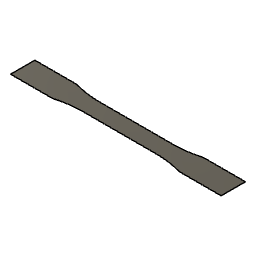
specimen_plastic_tensile_testing v3 (Autodesk Fusion 360 design; units mm, degrees)
Autodesk Fusion 360 part; units mm, degrees
sketch "Esquisse1" plane through (0, 0, 0) normal (0, 0, 1) x (1, 0, 0)
  line L0 (-28.5, 6.5) -> (0, 6.5)
  line L1 (0, 6.5) -> (0, 0) construction
  line L2 (0, 0) -> (-35.4205, 0) construction
  line L3 (-82.5, 9.5) -> (-49.6424, 9.5)
  line L4 (-35.4205, 0) -> (-82.5, 0) construction
  line L5 (-82.5, 0) -> (-82.5, 9.5)
  arc A0 (-49.6424, 9.5) -> (-28.5, 6.5) centre (-28.5, 82.5) ccw
  line L6 (-28.5, -6.5) -> (0, -6.5)
  arc A1 (-28.5, -6.5) -> (-49.6424, -9.5) centre (-28.5, -82.5) ccw
  line L7 (-82.5, -9.5) -> (-49.6424, -9.5)
  line L8 (-82.5, 0) -> (-82.5, -9.5)
  arc A2 (49.6424, -9.5) -> (28.5, -6.5) centre (28.5, -82.5) ccw
  line L9 (28.5, -6.5) -> (0, -6.5)
  line L10 (82.5, -9.5) -> (49.6424, -9.5)
  line L11 (82.5, 0) -> (82.5, -9.5)
  line L12 (82.5, 0) -> (82.5, 9.5)
  line L13 (82.5, 9.5) -> (49.6424, 9.5)
  arc A3 (28.5, 6.5) -> (49.6424, 9.5) centre (28.5, 82.5) ccw
  line L14 (28.5, 6.5) -> (0, 6.5)
  dimension "d1" = 28.5
  dimension "d9" = 6.5
  dimension "d10" = 152
  dimension "d13" = 82.5
  dimension "d14" = 9.5
  constraint horizontal L0
  constraint vertical L1
  constraint horizontal L2
  constraint coincident L1.end L2.start
  constraint horizontal L3
  constraint horizontal L4
  constraint vertical L5
  constraint coincident L1.end L4
  constraint tangent L0 A0
  constraint symmetric L0.start L4 L6.start
  constraint symmetric L0.end L4 L6.end
  constraint symmetric L3.start L4 L7.start
  constraint symmetric L3.end L4 A1.end
  constraint symmetric L5.start L4 L8.start
  constraint symmetric L4 A0 A1
  constraint symmetric L0.start L1 A3.start
  constraint symmetric L0.end L1 L14.end
  constraint symmetric L1 L3.start L12.end
  constraint symmetric L1 L3.end L13.end
  constraint symmetric L1 L4.end L11.start
  constraint symmetric L1 A0 A3
  constraint symmetric L1 L6.start A2.end
  constraint symmetric L1 L6.end L9.end
  constraint symmetric L1 A1.end A2.start
  constraint symmetric L1 A1 A2
  constraint symmetric L1 L7.start L10.start
  measures "d1" distance of L0.start L0.end
  measures "d9" distance of L0 L2
  measures "d10" diameter of A0
  measures "d13" distance of L1 L5
  measures "d14" distance of L3.start L4.end
extrude "Extrusion1" add sketch "Esquisse1" along normal blind 0.28
equation "d1 = Ln / 2"
equation "Wn = 13 mm" comment "Width of narrow section"
equation "Ln = 57 mm" comment "Length of narrow section"
equation "Wo = 19 mm" comment "Width overall, min"
equation "Lo = 165 mm" comment "Length overall, min"
equation "Dg = 10 mm" comment "Distance between grips"
equation "Rf = 76 mm" comment "Radius of fillet"
equation "d9 = Wn / 2"
equation "d10 = Rf * 2"
equation "d13 = Lo / 2"
equation "d14 = Wo / 2"
equation "To = 0.28 mm" comment "Thickness"
equation "d16 = To"
